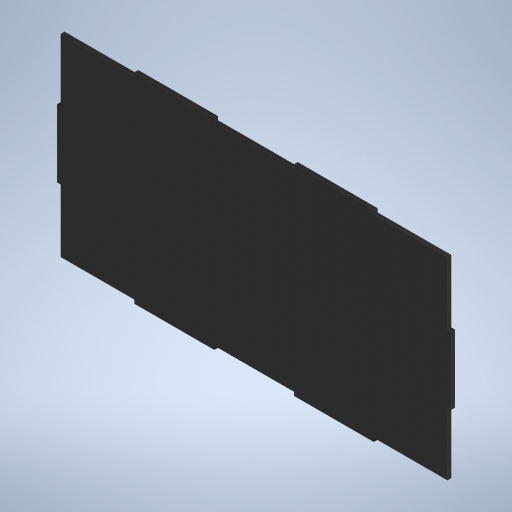
# Autodesk Inventor part: Final Product backplate
Saved by Autodesk Inventor 2024 (Build 280153000, 153)
## iProperties
Created: 2024-02-22
Part Number: Final Product backplate
Material: Generic
Document SubType Name: Modeling
Designer: flynf
Density: 1 g/cm^3
Appearance: Black Cast
Author: flynf
Autodesk Inventor part; units mm, degrees
ref_plane "YZ Plane" through (0, 0, 0) normal (1, 0, 0) x (0, 1, 0)
ref_plane "XZ Plane" through (0, 0, 0) normal (0, 1, 0) x (-1, 0, 0)
ref_plane "XY Plane" through (0, 0, 0) normal (0, 0, 1) x (1, 0, 0)
sketch "Sketch1" plane through (0, 0, 0) normal (0, 0, 1) x (1, 0, 0)
  line L0 (0, 0) -> (-2032, 0)
  line L1 (-2032, 0) -> (-2032, 1016)
  line L2 (-2032, 1016) -> (0, 1016)
  line L3 (0, 1016) -> (0, 0)
  line L4 (19.05, 1035.05) -> (-2051.05, 1035.05)
  line L5 (-2051.05, 1035.05) -> (-2051.05, -19.05)
  line L6 (-2051.05, -19.05) -> (19.05, -19.05)
  line L7 (19.05, -19.05) -> (19.05, 1035.05)
  line L8 (-1644.65, 1016) -> (-1644.65, 1035.05)
  line L9 (-1225.55, 1016) -> (-1225.55, 1035.05)
  line L10 (-806.45, 1016) -> (-806.45, 1035.05)
  line L11 (-387.35, 1016) -> (-387.35, 1035.05)
  line L12 (-1644.65, -19.05) -> (-1644.65, 0)
  line L13 (-1225.55, -19.05) -> (-1225.55, 0)
  line L14 (-806.45, -19.05) -> (-806.45, 0)
  line L15 (-387.35, -19.05) -> (-387.35, 0)
  line L16 (0, 330.2) -> (19.05, 330.2)
  line L17 (0, 685.8) -> (19.05, 685.8)
  line L18 (-2032, 685.8) -> (-2051.05, 685.8)
  line L19 (-2032, 330.2) -> (-2051.05, 330.2)
  point P0 (-1644.65, 0)
  point P1 (-1225.55, 0)
  point P2 (-806.45, 0)
  point P3 (-387.35, 0)
  dimension "d0" = 2032
  dimension "d1" = 1016
  dimension "d2" = 19.05
  dimension "d3" = 406.4
  dimension "d4" = 419.1
  dimension "d5" = 419.1
  dimension "d6" = 419.1
  dimension "d7" = 419.1
  dimension "d8" = 419.1
  dimension "d9" = 419.1
  dimension "d10" = 349.25
  dimension "d11" = 349.25
  dimension "d12" = 355.6
  dimension "d13" = 406.4
  dimension "d14" = 349.25
  dimension "d15" = 349.25
  constraints: 40 end point, 16 point on line, 8 parallel, 7 perpendicular, 2 horizontal, 3 other
  measures "d0" distance of L1.end L2.end
  measures "d1" distance of L0.end L1.end
  measures "d2" distance between parallel lines of L2 L4
  measures "d3" distance between parallel lines of L5 L8
  measures "d4" distance between parallel lines of L9 L8
  measures "d5" distance between parallel lines of L10 L9
  measures "d6" distance between parallel lines of L11 L10
  measures "d7" distance between parallel lines of L13 L12
  measures "d8" distance between parallel lines of L14 L13
  measures "d9" distance between parallel lines of L15 L14
  measures "d10" distance between parallel lines of L16 L6
  measures "d11" distance between parallel lines of L4 L17
  measures "d12" distance between parallel lines of L17 L16
  measures "d13" distance between parallel lines of L5 L12
  measures "d14" distance between parallel lines of L4 L18
  measures "d15" distance between parallel lines of L6 L19
extrude "Extrusion1" add sketch "Sketch1" along normal blind 19.05 contours L0 L1 L2 L3 | L15 L6 L14 L0 | L3 L17 L7 L16 | L13 L6 L12 L0 | L2 L10 L4 L11 | L19 L5 L18 L1 | L2 L8 L4 L9
body "Solid1"
